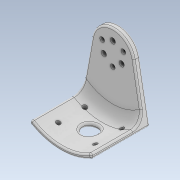
# Autodesk Inventor part: thigh_hip_connector
Saved by Autodesk Inventor 2020 (Build 240168000, 168)
## iProperties
Created: 2021-01-06
Part Number: thigh_hip_connector
Material: Generic
Document SubType Name: Modeling
Designer: DELL
Density: 1 g/cm^3
Appearance: Clear - Blue
Author: DELL
Autodesk Inventor part; units mm, degrees
ref_plane "YZ Plane" through (0, 0, 0) normal (1, 0, 0) x (0, 1, 0)
ref_plane "XZ Plane" through (0, 0, 0) normal (0, 1, 0) x (-1, 0, 0)
ref_plane "XY Plane" through (0, 0, 0) normal (0, 0, 1) x (1, 0, 0)
sketch "Sketch1" plane through (0, 0, 0) normal (0, 0, 1) x (1, 0, 0)
  circle A0 centre (0, 0) radius 20
  line L0 (-19.68, 3.5636) -> (-29, -47.9062)
  line L1 (19.68, 3.5636) -> (29, -47.9062)
  line L2 (9.9593, -5.75) -> (0, 0) construction
  circle A1 centre (8.4134, -4.8575) radius 2.5
  line L3 (0, 0) -> (9.9593, 5.75) construction
  line L4 (0, 0) -> (-9.9593, -5.75) construction
  circle A2 centre (-8.4134, -4.8575) radius 2.5
  circle A3 centre (0, 0) radius 9.715 construction
  circle A4 centre (0, 0) radius 11.5 construction
  circle A5 centre (0, 9.715) radius 2.5
  line L5 (0, 0) -> (-9.9593, 5.75) construction
  line L6 (11.5, 0) -> (-11.5, 0) construction
  circle A6 centre (-9.9593, 5.75) radius 4
  circle A7 centre (-9.9593, 5.75) radius 2.25
  line L7 (0, -48.5721) -> (0, 22.5) construction
  circle A8 centre (0, -11.5) radius 2.25
  circle A9 centre (0, -11.5) radius 4
  circle A10 centre (9.9593, 5.75) radius 4
  circle A11 centre (9.9593, 5.75) radius 2.25
  arc A12 (-28.2326, -43.6683) -> (28.2326, -43.6683) centre (0, 0) ccw
  arc A13 (-29, -47.9062) -> (29, -47.9062) centre (0, 0) ccw
  line L8 (8, -59.5) -> (-8, -59.5)
  line L9 (-8, -59.5) -> (-8, -52.5)
  line L10 (-8, -52.5) -> (8, -52.5)
  line L11 (8, -52.5) -> (8, -59.5)
  line L12 (8, -59.5) -> (-8, -52.5) construction
  line L13 (-8, -59.5) -> (8, -52.5) construction
  point P0 (0, 11.4686)
  point P1 (0, 11.4686)
  point P2 (11.5, 0)
  point P3 (-11.5, 0)
  point P4 (0, -56)
  dimension "d18" = 23
  dimension "d0" = 40
  dimension "d17" = 19.43
  dimension "d19" = 30
  dimension "d20" = 30
  dimension "d21" = 4.5
  dimension "d22" = 8
  dimension "d23" = 5
  dimension "d24" = 104
  dimension "d25" = 112
  dimension "d48" = 58
  dimension "d60" = 16
  dimension "d61" = 7
  constraints: 26 end point, 13 centre point, 10 coincident, 10 point on circle, 8 point on line, 6 equal radius, 2 midpoint, 2 parallel, 2 tangent, 1 horizontal, 1 perpendicular, 1 vertical, 17 other
  measures "d0" diameter of A0
  measures "d17" diameter of A3
  measures "d19" angle to the sketch x axis of L5
  measures "d20" angle to the sketch x axis of L4
  measures "d21" diameter of A11
  measures "d22" diameter of A10
  measures "d23" diameter of A5
  measures "d24" diameter of A12
  measures "d25" diameter of A13
  measures "d48" distance of L1.end L0.end
  measures "d60" distance of L8.start L8.end
  measures "d61" distance of L8.end L9.end
extrude "Extrusion1" add sketch "Sketch1" along normal blind 6 contours A0 | A0 L1 A12 L0 | L1 A13 L11 L10 L9 L0 A12 | A13 L9 L10 L11 | A1 | A2 | A5 | A6 | A9 | A10
extrude "Extrusion2" cut sketch "Sketch1" along normal blind 3.5 contours A6 | A9 | A10 | A11
extrude "Extrusion3" cut sketch "Sketch1" along normal through all contours A1 | A2 | A5
extrude "Extrusion4" add sketch "Sketch1" along normal blind 49 from surface at 6 contours L1 A13 L11 L10 L9 L0 A12 | A13 L9 L10 L11
extrude "Extrusion8" add sketch "Sketch1" along normal blind 15 contours L11 L8 L9 A13 | A13 L9 L10 L11
fillet "Fillet1" radius 10 1 edges at (0, -52, 6)
fillet "Fillet2" radius 1.5 27 edges at (-18.8782, -52.722, 0) (18.8782, -52.722, 0) (0, -56, 55) (29, -47.9062, 27.5) (-29, -47.9062, 27.5) (-24.34, -22.1713, 0) (24.34, -22.1713, 0) (0, 20, 0) (-22.9703, -14.6071, 6) (-27.6237, -40.3053, 8.7268) (-28.2326, -43.6683, 35.5) (22.9703, -14.6071, 6) (27.6237, -40.3053, 8.7268) (28.2326, -43.6683, 35.5) (0, 20, 6) (0, -52, 55) (-28.6163, -45.7872, 55) (28.6163, -45.7872, 55) (0, -56, 15) (8, -57.4628, 15) (8, -59.5, 7.5) (0, -59.5, 15) (-8, -57.4628, 15) (-8, -59.5, 7.5) (8, -57.4628, 0) (-8, -57.4628, 0) (0, -59.5, 0)
sketch "Sketch2" plane through (0, 0, 0) normal (0, 1, 0) x (-1, 0, 0)
  line L0 (-28.6245, 0) -> (-28.6245, 55) construction
  line L1 (18.204, 0) -> (-18.204, 0) construction
  line L2 (27.1485, 55) -> (-27.1485, 55) construction
  line L3 (-28.6245, 27.5) -> (28.8142, 27.5) construction
  line L4 (28.8142, 53.5) -> (28.8142, 1.5) construction
  line L5 (-28.6245, 53.5) -> (-28.6245, 16) construction
  line L6 (0, 0) -> (0, 55) construction
  circle A0 centre (0, 27.5) radius 7
  circle A1 centre (0, 27.5) radius 25
  line L7 (-17.5, 40) -> (17.5, 40) construction
  line L8 (17.5, 40) -> (17.5, 15) construction
  line L9 (17.5, 15) -> (-17.5, 15) construction
  line L10 (-17.5, 15) -> (-17.5, 40) construction
  line L11 (-17.5, 40) -> (17.5, 15) construction
  line L12 (17.5, 40) -> (-17.5, 15) construction
  circle A2 centre (17.5, 15) radius 2
  circle A3 centre (17.5, 15) radius 1.25
  circle A4 centre (-17.5, 15) radius 2
  circle A5 centre (-17.5, 15) radius 1.25
  circle A6 centre (17.5, 40) radius 2
  circle A7 centre (17.5, 40) radius 1.25
  circle A8 centre (-17.5, 40) radius 2
  circle A9 centre (-17.5, 40) radius 1.25
  dimension "d40" = 14
  dimension "d41" = 50
  dimension "d50" = 25
  dimension "d51" = 35
  dimension "d52" = 2.5
  dimension "d53" = 4
  constraints: 18 end point, 10 centre point, 6 coincident, 6 midpoint, 6 symmetric about line, 2 parallel, 2 point on line, 1 collinear, 1 horizontal, 1 perpendicular, 1 vertical, 6 other
  measures "d40" diameter of A0
  measures "d41" diameter of A1
  measures "d50" distance of L7.end L8.end
  measures "d51" distance of L8.end L9.end
  measures "d52" diameter of A3
  measures "d53" diameter of A2
extrude "Extrusion5" cut sketch "Sketch2" against normal through all contours A0 | A3 | A5 | A7 | A9
extrude "Extrusion6" cut sketch "Sketch2" against normal blind 51 contours A2 | A3 | A4 | A5 | A6 | A7 | A8 | A9
fillet "Fillet4" radius 2 2 edges at (7, -51.5267, 27.5178) (7, -55.5608, 27.5023)
body "Solid1"
